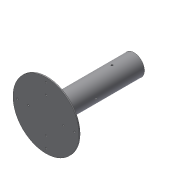
# Autodesk Inventor part: Pole Base
Saved by Autodesk Inventor 2015 SP1 (Build 190203100, 203)
## iProperties
Created: 2015-08-24
Part Number: Pole Base
Material: 一般
Document SubType Name: Modeling
Designer: nobuhiro
Density: 1 g/cm^3
Appearance: 既定
Author: nobuhiro
Autodesk Inventor part; units mm, degrees
ref_plane "YZ Plane" through (0, 0, 0) normal (1, 0, 0) x (0, 1, 0)
ref_plane "XZ Plane" through (0, 0, 0) normal (0, 1, 0) x (-1, 0, 0)
ref_plane "XY Plane" through (0, 0, 0) normal (0, 0, 1) x (1, 0, 0)
sketch "スケッチ1" plane through (0, 0, 0) normal (0, 0, 1) x (1, 0, 0)
  line L0 (0, 0) -> (150, 0)
  line L1 (150, 0) -> (150, 5)
  line L2 (150, 5) -> (0, 5)
  line L3 (0, 5) -> (0, 0)
  line L4 (42.5, 0) -> (47.5, 0)
  line L5 (47.5, 0) -> (47.5, 500)
  line L6 (47.5, 500) -> (42.5, 500)
  line L7 (42.5, 500) -> (42.5, 0)
  dimension "d1" = 47.5
  dimension "d2" = 150
  dimension "d3" = 5
  dimension "d4" = 5
  dimension "d5" = 500
  constraints: 16 end point, 4 parallel, 2 horizontal, 2 perpendicular, 1 point on line
  measures "d1" distance between parallel lines of L3 L5
  measures "d2" distance between parallel lines of L3 L1
  measures "d3" distance of L0.end L1.end
  measures "d4" distance of L5.end L6.end
  measures "d5" distance between parallel lines of L0 L6
revolve "回転1" add sketch "スケッチ1" angle 360 about axis through (0, 5, 0) along (0, -1, 0)
sketch "スケッチ2" plane through (0, 0, 0) normal (0, -1, 0) x (1, 0, 0)
  circle A0 centre (0, 0) radius 150 projected
  circle A1 centre (0, 130) radius 4
  circle A2 centre (0, 80) radius 4
  circle A3 centre (-130, 0) radius 4
  circle A4 centre (-80, 0) radius 4
  circle A5 centre (0, -130) radius 4
  circle A6 centre (0, -80) radius 4
  circle A7 centre (130, 0) radius 4
  circle A8 centre (80, 0) radius 4
  dimension "d7" = 8
  dimension "d8" = 130
  dimension "d9" = 80
  dimension "d12" = 360
  constraints: 8 centre point, 2 vertical alignment, 1 equal radius, 17 other
  measures "d7" diameter of A1
  measures "d8" distance of A1.centre A0.centre
  measures "d9" distance of A0.centre A2.centre
extrude "押し出し1" cut sketch "スケッチ2" against normal through all keep common part
sketch "スケッチ3" plane through (0, 0, 0) normal (0, 0, 1) x (1, 0, 0)
  circle A0 centre (0, 50) radius 6
  circle A1 centre (0, 300) radius 6
  line L0 (-150, 0) -> (150, 0) projected
  point P0 (0, 0)
  dimension "d16" = 12
  dimension "d17" = 50
  dimension "d18" = 300
  constraints: 2 centre point, 2 vertical alignment, 1 equal radius
  measures "d16" diameter of A0
  measures "d17" distance from line of A0.centre L0
  measures "d18" distance from line of L0 A1.centre
extrude "押し出し2" cut sketch "スケッチ3" along normal through all both and the other way through all
sketch "スケッチ4" plane through (0, 0, 0) normal (1, 0, 0) x (0, 1, 0)
  circle A0 centre (180, 0) radius 6
  line L0 (0, 4) -> (0, -4) projected
  point P0 (0, 0)
  dimension "d21" = 12
  dimension "d22" = 180
  constraints: 1 centre point
  measures "d21" diameter of A0
  measures "d22" distance from line of L0 A0.centre
extrude "押し出し3" cut sketch "スケッチ4" along normal through all both and the other way through all
